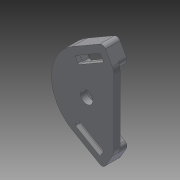
# Autodesk Inventor part: WireOrganizer
Saved by Autodesk Inventor 2015 (Build 190159000, 159)
## iProperties
Created: 2014-12-12
Part Number: WireOrganizer
Material: Generic
Document SubType Name: Modeling
Designer: rawrdong
Density: 1 g/cm^3
Appearance: Default
Author: rawrdong
Autodesk Inventor part; units mm, degrees
ref_plane "YZ Plane" through (0, 0, 0) normal (1, 0, 0) x (0, 1, 0)
ref_plane "XZ Plane" through (0, 0, 0) normal (0, 1, 0) x (-1, 0, 0)
ref_plane "XY Plane" through (0, 0, 0) normal (0, 0, 1) x (1, 0, 0)
sketch "Sketch1" plane through (0, 0, 0) normal (0, 1, 0) x (-1, 0, 0)
  line L0 (46.641819, 0) -> (-23.320909, -40.393) construction
  line L1 (-23.320909, -40.393) -> (-23.320909, 40.393) construction
  line L2 (-23.320909, 40.393) -> (46.641819, 0) construction
  line L3 (46.841819, 0.11547) -> (31.91539, -8.502308)
  line L4 (31.91539, 8.733248) -> (46.841819, 0.11547)
  line L5 (56.841819, 0.11547) -> (34.41539, -12.832435)
  line L6 (34.41539, 13.063375) -> (56.841819, 0.11547)
  circle A0 centre (38.45, 0) radius 1.5
  line L7 (-41.958879, -51.153637) -> (-41.11627, -50.667156)
  line L8 (-31.932835, 45.365097) -> (-31.906279, 45.580706)
  line L9 (33.672922, 9.046442) -> (40.601125, 5.046442)
  line L10 (40.601125, 5.046442) -> (41.951125, 7.38471)
  line L11 (41.951125, 7.38471) -> (35.022922, 11.38471)
  line L12 (35.022922, 11.38471) -> (33.672922, 9.046442)
  line L13 (33.672922, 9.046442) -> (41.951125, 7.38471) construction
  line L14 (40.601125, 5.046442) -> (35.022922, 11.38471) construction
  line L15 (34.41539, 13.063375) -> (31.91539, 8.733248)
  line L16 (31.91539, -8.502308) -> (34.41539, -12.832435)
  line L17 (31.91539, -8.502308) -> (31.91539, 8.733248)
  line L18 (39.062024, 10.38064) -> (36.562024, 6.050513) construction
  line L19 (38.45, 0) -> (14.580023, 0) construction
  line L20 (33.672922, -9.046442) -> (40.601125, -5.046442)
  line L21 (40.601125, -5.046442) -> (41.951125, -7.38471)
  line L22 (41.951125, -7.38471) -> (35.022922, -11.38471)
  line L23 (35.022922, -11.38471) -> (33.672922, -9.046442)
  point P0 (0, 0)
  point P1 (0, 0)
  point P2 (37.812024, 8.215576)
  point P3 (-23.320909, 0)
  dimension "d0" = 80.786
  dimension "d1" = 0.2
  dimension "d2" = 3
  dimension "d3" = 38.45
  dimension "d4" = 2.7
  dimension "d5" = 5
  dimension "d6" = 5
  dimension "d7" = 8
  dimension "d8" = 0
  dimension "d29" = 1.25
  constraints: 48 end point, 6 point on line, 4 midpoint, 4 parallel, 4 perpendicular, 4 symmetric about line, 2 horizontal alignment, 1 centre point, 1 coincident, 1 collinear, 1 horizontal, 1 vertical, 7 other
  measures "d0" distance of L0.start L0.end
  measures "d1" distance between parallel lines of L2 L4
  measures "d2" diameter of A0
  measures "d3" distance of L19.start point (0, 0)
  measures "d4" distance between parallel lines of L9 L11
  measures "d5" distance between parallel lines of L5 L3
  measures "d6" distance between parallel lines of L4 L6
  measures "d7" distance of L10.end L11.end
  measures "d8" distance between parallel lines of L0 L3
  measures "d29" distance between parallel lines of L16 L23
extrude "Extrusion1" add sketch "Sketch1" along normal blind 2 contours L4 L15 L6 L5 L16 L3
fillet "Fillet1" radius 5 1 edges at (-46.8418, 1, 0.1155)
fillet "Fillet2" radius 10 1 edges at (-56.8418, 1, 0.1155)
fillet "Fillet3" radius 0.5 8 edges at (-33.6729, 1, 9.0464) (-35.0229, 1, 11.3847) (-41.9511, 1, 7.3847) (-40.6011, 1, 5.0464) (-35.0229, 1, -11.3847) (-41.9511, 1, -7.3847) (-40.6011, 1, -5.0464) (-33.6729, 1, -9.0464)
sketch "Sketch2" plane through (0, 0, 0) normal (0, -1, 0) x (1, 0, 0)
  arc A0 (-41.841819, 8.775724) -> (-41.841819, -8.544784) centre (-36.841819, 0.11547) ccw
  line L0 (-34.41539, -12.832435) -> (-41.841819, -8.544784)
  line L1 (-31.91539, -8.502308) -> (-34.41539, -12.832435)
  line L2 (-39.341819, -4.214657) -> (-31.91539, -8.502308)
  arc A1 (-39.341819, 4.445597) -> (-39.341819, -4.214657) centre (-36.841819, 0.11547) ccw
  line L3 (-31.91539, 8.733248) -> (-39.341819, 4.445597)
  line L4 (-34.41539, 13.063375) -> (-31.91539, 8.733248)
  line L5 (-41.841819, 8.775724) -> (-34.41539, 13.063375)
  line L6 (-34.772922, 10.951698) -> (-33.922922, 9.479455)
  arc A2 (-34.105935, 8.796442) -> (-33.922922, 9.479455) centre (-34.355935, 9.229455) ccw
  line L7 (-34.105935, 8.796442) -> (-40.168112, 5.296442)
  arc A3 (-40.851125, 5.479455) -> (-40.168112, 5.296442) centre (-40.418112, 5.729455) ccw
  line L8 (-40.851125, 5.479455) -> (-41.701125, 6.951698)
  arc A4 (-41.518112, 7.63471) -> (-41.701125, 6.951698) centre (-41.268112, 7.201698) ccw
  line L9 (-41.518112, 7.63471) -> (-35.455935, 11.13471)
  arc A5 (-34.772922, 10.951698) -> (-35.455935, 11.13471) centre (-35.205935, 10.701698) ccw
  line L10 (-35.455935, -11.13471) -> (-41.518112, -7.63471)
  arc A6 (-41.701125, -6.951698) -> (-41.518112, -7.63471) centre (-41.268112, -7.201698) ccw
  line L11 (-41.701125, -6.951698) -> (-40.851125, -5.479455)
  arc A7 (-40.168112, -5.296442) -> (-40.851125, -5.479455) centre (-40.418112, -5.729455) ccw
  line L12 (-40.168112, -5.296442) -> (-34.105935, -8.796442)
  arc A8 (-33.922922, -9.479455) -> (-34.105935, -8.796442) centre (-34.355935, -9.229455) ccw
  line L13 (-33.922922, -9.479455) -> (-34.772922, -10.951698)
  arc A9 (-35.455935, -11.13471) -> (-34.772922, -10.951698) centre (-35.205935, -10.701698) ccw
  line L14 (-31.91539, 8.733248) -> (-31.91539, -8.502308)
  circle A10 centre (-38.45, 0) radius 1.5
  point P0 (0, 0)
  dimension "d17" = 38.45
  dimension "d18" = 3
  constraints: 2 end point, 1 centre point, 1 horizontal alignment, 1 vertical
  measures "d17" distance of point (0, 0) A10.centre
  measures "d18" diameter of A10
extrude "Extrusion2" add sketch "Sketch2" along normal blind 1.5
fillet "Fillet4" radius 1 2 edges at (-34.4154, 0.25, 13.0634) (-34.4154, 0.25, -12.8324)
fillet "Fillet5" radius 3 2 edges at (-31.9154, -0.75, 8.7332) (-31.9154, -0.75, -8.5023)
fillet "Fillet6" radius 1 2 edges at (-32.0104, 1, 8.6784) (-32.0104, 1, -8.4475)
shell "Shell1" thickness 1.25 removed faces 1 at (-42.355693, 2, -4.49705)
fillet "Fillet7" radius 0.5 3 edges at (-41.4618, 0.875, 4.3248) (-41.329, 0.875, -4.2352) (-42.7765, 0.875, -6.3143)
chamfer "Chamfer2" distance 0.5 angle 45 16 edges at (-38.487, 2, 9.3847) (-41.7511, 2, 7.3311) (-41.2761, 2, 6.2156) (-40.5475, 2, 5.2465) (-37.137, 2, 7.0464) (-33.873, 2, 9.1) (-34.3479, 2, 10.2156) (-35.0765, 2, 11.1847) (-37.137, 2, -7.0464) (-40.5475, 2, -5.2465) (-41.2761, 2, -6.2156) (-41.7511, 2, -7.3311) (-38.487, 2, -9.3847) (-35.0765, 2, -11.1847) (-34.3479, 2, -10.2156) (-33.873, 2, -9.1)
sketch "Sketch3" plane through (0, -1.5, 0) normal (0, -1, 0) x (1, 0, 0)
  circle A0 centre (-38.45, 0) radius 1.5
  arc A1 (-34.105935, 8.796442) -> (-33.922922, 9.479455) centre (-34.355935, 9.229455) ccw
  line L0 (-34.105935, 8.796442) -> (-40.168112, 5.296442)
  arc A2 (-40.851125, 5.479455) -> (-40.168112, 5.296442) centre (-40.418112, 5.729455) ccw
  line L1 (-40.851125, 5.479455) -> (-41.701125, 6.951698)
  arc A3 (-41.518112, 7.63471) -> (-41.701125, 6.951698) centre (-41.268112, 7.201698) ccw
  line L2 (-41.518112, 7.63471) -> (-35.455935, 11.13471)
  arc A4 (-34.772922, 10.951698) -> (-35.455935, 11.13471) centre (-35.205935, 10.701698) ccw
  line L3 (-34.772922, 10.951698) -> (-33.922922, 9.479455)
  arc A5 (-41.701125, -6.951698) -> (-41.518112, -7.63471) centre (-41.268112, -7.201698) ccw
  line L4 (-41.701125, -6.951698) -> (-40.851125, -5.479455)
  arc A6 (-40.168112, -5.296442) -> (-40.851125, -5.479455) centre (-40.418112, -5.729455) ccw
  line L5 (-40.168112, -5.296442) -> (-34.105935, -8.796442)
  arc A7 (-33.922922, -9.479455) -> (-34.105935, -8.796442) centre (-34.355935, -9.229455) ccw
  line L6 (-33.922922, -9.479455) -> (-34.772922, -10.951698)
  arc A8 (-35.455935, -11.13471) -> (-34.772922, -10.951698) centre (-35.205935, -10.701698) ccw
  line L7 (-35.455935, -11.13471) -> (-41.518112, -7.63471)
  arc A9 (-32.317314, -9.19846) -> (-31.91539, -7.69846) centre (-34.91539, -7.69846) ccw
  line L8 (-31.91539, -7.69846) -> (-31.91539, 7.9294)
  arc A10 (-31.91539, 7.9294) -> (-32.317314, 9.4294) centre (-34.91539, 7.9294) ccw
  line L9 (-32.317314, 9.4294) -> (-33.91539, 12.197349)
  arc A11 (-33.91539, 12.197349) -> (-35.281416, 12.563375) centre (-34.781416, 11.697349) ccw
  line L10 (-35.281416, 12.563375) -> (-41.841819, 8.775724)
  arc A12 (-41.841819, 8.775724) -> (-41.841819, -8.544784) centre (-36.841819, 0.11547) ccw
  line L11 (-41.841819, -8.544784) -> (-35.281416, -12.332435)
  arc A13 (-35.281416, -12.332435) -> (-33.91539, -11.966409) centre (-34.781416, -11.466409) ccw
  line L12 (-33.91539, -11.966409) -> (-32.317314, -9.19846)
  line L13 (-40.418112, 5.729455) -> (-34.355935, 9.229455)
  line L14 (-34.355935, 9.229455) -> (-35.205935, 10.701698)
  line L15 (-35.205935, 10.701698) -> (-41.268112, 7.201698)
  line L16 (-41.268112, 7.201698) -> (-40.418112, 5.729455)
  line L17 (-34.355935, -9.229455) -> (-40.418112, -5.729455)
  line L18 (-40.418112, -5.729455) -> (-41.268112, -7.201698)
  line L19 (-41.268112, -7.201698) -> (-35.205935, -10.701698)
  line L20 (-35.205935, -10.701698) -> (-34.355935, -9.229455)
  point P0 (0, 0)
  dimension "d30" = 0.5
  dimension "d31" = 0.5
  constraints: 16 end point, 6 other
  measures "d30" distance between parallel lines of L0 L13
  measures "d31" distance between parallel lines of L5 L17
extrude "Extrusion3" add sketch "Sketch3" against normal blind 1 contours L0 A2 L1 A3 L2 A4 L3 A1 | L4 A6 L5 A7 L6 A8 L7 A5
fillet "Fillet8" radius 0.25 8 edges at (-35.2059, -1, 10.7017) (-34.3559, -1, 9.2295) (-41.2681, -1, 7.2017) (-40.4181, -1, 5.7295) (-35.2059, -1, -10.7017) (-34.3559, -1, -9.2295) (-40.4181, -1, -5.7295) (-41.2681, -1, -7.2017)
fillet "Fillet9" radius 0.25 1 edges at (-42.8576, 0.875, 6.4695)
body "Solid1"
